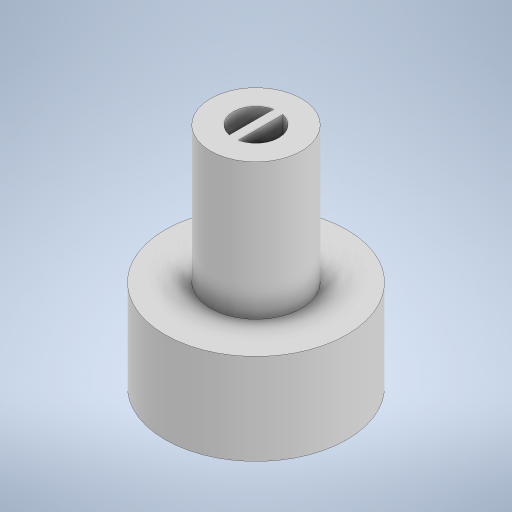
# Autodesk Inventor part: pot başlık
Saved by Autodesk Inventor 2023 (Build 270158000, 158)
## iProperties
Created: 2023-03-11
Part Number: pot başlık
Material: Generic
Document SubType Name: Modeling
Designer: Umut Yücesoy
Density: 1 g/cm^3
Appearance: Default
Author: Umut Yücesoy
Autodesk Inventor part; units mm, degrees
ref_plane "YZ Plane" through (0, 0, 0) normal (1, 0, 0) x (0, 1, 0)
ref_plane "XZ Plane" through (0, 0, 0) normal (0, 1, 0) x (-1, 0, 0)
ref_plane "XY Plane" through (0, 0, 0) normal (0, 0, 1) x (1, 0, 0)
sketch "Sketch1" plane through (0, 0, 0) normal (0, 1, 0) x (-1, 0, 0)
  circle A0 centre (0, 0) radius 5
  dimension "d1" = 10
  constraints: 1 centre point
  measures "d1" diameter of A0
extrude "Extrusion1" add sketch "Sketch1" along normal blind 15
sketch "Sketch2" plane through (0, 15, 0) normal (0, 1, 0) x (1, 0, 0)
  circle A0 centre (0, 0) radius 2.5
  line L0 (0, 0) -> (-0.5, 0)
  line L1 (-0.5, 0) -> (-0.5, -2.4495)
  line L2 (-0.5, 0) -> (-0.5, 2.4495)
  line L3 (0, 0) -> (0, 2.5)
  line L4 (0.5, 0) -> (0.5, -2.4495)
  line L5 (0.5, 0) -> (0.5, 2.4495)
  dimension "d4" = 5
  dimension "d5" = 0.5
  constraints: 12 end point, 4 symmetric about line, 2 point on circle, 2 vertical, 1 centre point, 1 coincident, 1 horizontal
  measures "d4" diameter of A0
  measures "d5" distance of L0.start L0.end
extrude "Extrusion2" cut sketch "Sketch2" against normal blind 10 contours A0 L4 L5 | A0 L2 L1
sketch "Sketch3" plane through (0, 0, 0) normal (0, -1, 0) x (1, 0, 0)
  circle A0 centre (0, 0) radius 10
  dimension "d8" = 20
  constraints: 1 centre point, 1 coincident
  measures "d8" diameter of A0
extrude "Extrusion3" add sketch "Sketch3" along normal blind 10
sketch "Sketch5" plane through (0, -10, 0) normal (0, -1, 0) x (1, 0, 0)
  circle A0 centre (0, 0) radius 2.5
  constraints: 1 centre point, 1 coincident
extrude "Extrusion4" cut sketch "Sketch5" against normal blind 5
sketch "Sketch6" plane through (0, 0, 0) normal (0, 0, 1) x (1, 0, 0)
  line L0 (-10, -10) -> (10, -10) projected
  line L1 (10, -10) -> (8, -10)
  line L2 (8, -10) -> (8, -5)
  line L3 (2.5359, -10) -> (4.5359, -10)
  line L4 (4.5359, -10) -> (4.5359, -5)
  line L5 (4.5359, -5) -> (8, -5)
  line L6 (8, -5) -> (4.5359, -7)
  line L7 (0, -15) -> (0, 20) projected
  point P0 (0, 0)
  dimension "d13" = 2
  dimension "d14" = 2
  dimension "d15" = 4
  dimension "d16" = 30
  dimension "d17" = 2
  constraints: 12 end point, 4 point on line, 3 perpendicular
  measures "d13" distance of L0.end L1.end
  measures "d14" distance of L3.start L3.end
  measures "d15" distance of L2.end L6.end
  measures "d16" angle of L6 L5
  measures "d17" distance from line of L0.end L2
revolve "Revolution1" cut sketch "Sketch6" angle 30 about axis through (0, -10, 0) along (0, -1, 0) contours L4 L6 L2 L0
pattern_circular "Circular Pattern1" count 6 over 360 about axis through (0, -10, 0) along (0, 1, 0) of "Revolution1"
body "Solid1"
